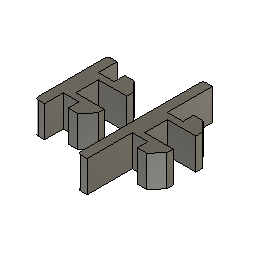
clips (Autodesk Fusion 360 design; units mm, degrees)
Autodesk Fusion 360 part; units mm, degrees
sketch "Esquisse1" plane through (0, 0, 0) normal (0, 0, 1) x (1, 0, 0)
  line L0 (4, -4.5) -> (2.5, -4.5)
  line L1 (2.5, -4.5) -> (2.5, -2.8)
  line L2 (2.5, -2.8) -> (0, -2.8)
  line L3 (0, -2.8) -> (0, 2.8)
  line L4 (0, 2.8) -> (2.5, 2.8)
  line L5 (2.5, 2.8) -> (2.5, 4.5)
  line L6 (5.5382, -2.8) -> (4, -4.5)
  line L7 (0, 5.8) -> (-1, 5.8)
  line L8 (-1.5, 5.3) -> (-1.5, -5.3)
  line L9 (-1, -5.8) -> (0, -5.8)
  line L10 (0, -5.8) -> (0, 5.8)
  line L11 (1.75, 0) -> (22.5, 0)
  line L12 (5.5382, 2.8) -> (4, 4.5)
  line L13 (4, 4.5) -> (2.5, 4.5)
  line L14 (1, 1.8) -> (5.5382, 1.8)
  line L15 (5.5382, -1.8) -> (1, -1.8)
  line L16 (1, -1.8) -> (1, 1.8)
  line L17 (5.5382, 2.8) -> (5.5382, 1.8)
  line L18 (5.5382, -1.8) -> (5.5382, -2.8)
  arc A0 (-1.5, -5.3) -> (-1, -5.8) centre (-1, -5.3) ccw
  arc A1 (-1, 5.8) -> (-1.5, 5.3) centre (-1, 5.3) ccw
  line L19 (10, -10) -> (11, -10)
  line L20 (11, -10) -> (11, 10)
  line L21 (11, 10) -> (10, 10)
  arc A2 (10, 10) -> (9.5, 9.5) centre (10, 9.5) ccw
  line L22 (9.5, 9.5) -> (9.5, -9.5)
  arc A3 (9.5, -9.5) -> (10, -10) centre (10, -9.5) ccw
  line L23 (16.5382, 2.8) -> (15, 4.5)
  line L24 (16.5382, 2.8) -> (16.5382, 1.8)
  line L25 (12, 1.8) -> (16.5382, 1.8)
  line L26 (12, -1.8) -> (12, 1.8)
  line L27 (16.5382, -1.8) -> (12, -1.8)
  line L28 (16.5382, -1.8) -> (16.5382, -2.8)
  line L29 (16.5382, -2.8) -> (15, -4.5)
  line L30 (15, -4.5) -> (13.5, -4.5)
  line L31 (13.5, -4.5) -> (13.5, -2.8)
  line L32 (13.5, -2.8) -> (11, -2.8)
  line L33 (11, -2.8) -> (11, 2.8)
  line L34 (13.5, 2.8) -> (13.5, 4.5)
  line L35 (15, 4.5) -> (13.5, 4.5)
  line L36 (11, 2.8) -> (13.5, 2.8)
  point P0 (-1.5, 5.8)
  dimension "d17" = 2.5
  dimension "d18" = 2.5
  dimension "d19" = 1.5
  dimension "d21" = 5.6
  dimension "d23" = 5.6
  dimension "d26" = 1.7
  dimension "d9" = 1.5
  dimension "d11" = 132.139
  dimension "d14" = 1
  dimension "d15" = 1
  dimension "d16" = 0.5
  dimension "d24" = 3
  dimension "d25" = 2.5
  dimension "d27" = 2.5
  dimension "d28" = 1.5
  dimension "d29" = 5.6
  dimension "d30" = 5.6
  dimension "d31" = 1.7
  dimension "d32" = 132.139
  dimension "d33" = 1
  dimension "d34" = 1
  dimension "d35" = 0.5
  dimension "d37" = 20
  constraint horizontal L4
  constraint perpendicular L4 L5
  constraint perpendicular L0 L17
  constraint perpendicular L0 L1
  constraint perpendicular L2 L17
  constraint perpendicular L3 L4
  constraint coincident origin L3
  constraint horizontal L7
  constraint vertical L8
  constraint horizontal L9
  constraint vertical L10
  constraint symmetric L7 L9 L11
  constraint symmetric L2 L4 L11
  constraint coincident origin L10
  constraint symmetric L6.start L11 L12.start
  constraint symmetric L0.start L11 L12.end
  constraint coincident L12.start L17.start
  constraint perpendicular L5 L13
  constraint horizontal L14
  constraint horizontal L15
  constraint vertical L16
  constraint symmetric L11 L14 L15
  constraint collinear L17 L18
  constraint tangent L8 A0
  constraint tangent L9 A0
  constraint coincident P0 L7
  constraint coincident P0 L8
  constraint tangent L7 A1
  constraint tangent L8 A1
  constraint equal A0 A1
  constraint horizontal L36
  constraint perpendicular L34 L36
  constraint perpendicular L24 L30
  constraint perpendicular L30 L31
  constraint perpendicular L24 L32
  constraint perpendicular L33 L36
  constraint horizontal L21
  constraint vertical L22
  constraint horizontal L19
  constraint vertical L20
  constraint coincident L23.start L24.start
  constraint perpendicular L34 L35
  constraint horizontal L25
  constraint horizontal L27
  constraint vertical L26
  constraint collinear L24 L28
  constraint tangent L22 A3
  constraint tangent L19 A3
  constraint tangent L21 A2
  constraint tangent A2 L22
  constraint equal A2 A3
  constraint symmetric L11 L19 L21
  constraint symmetric L11 L25 L27
  measures "d17" distance of L4.end L3.end
  measures "d18" distance of L1.end L2.end
  measures "d19" distance of L0.start L0.end
  measures "d21" distance of L2 L4
  measures "d23" distance of L12.start L6.start
  measures "d26" distance of L1.end L0.end
  measures "d9" distance of L7.start P0
  measures "d11" angle of L0 L6
  measures "d14" distance of L10 L16
  measures "d15" distance of L4 L14
  measures "d16" radius of A0
  measures "d24" distance of L4 L7.end
  measures "d25" distance of L33.end L34.start
  measures "d27" distance of L31.end L32.end
  measures "d28" distance of L30.end L29.end
  measures "d29" distance of L32 L36
  measures "d30" distance of L23.start L28.end
  measures "d31" distance of L31.end L30.end
  measures "d32" angle of L29 L30
  measures "d33" distance of L20 L26
  measures "d34" distance of L25 L36
  measures "d35" radius of A3
  measures "d37" distance of L19 L21
extrude "Extrusion1" add sketch "Esquisse1" along normal blind 5 makes body 1 at (-1.5, 1.7667, 1.6667) makes body 2 at (9.5, 3.1667, 1.6667)
